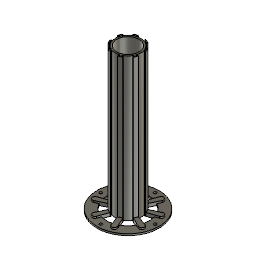
Wifi lamp assembly (Autodesk Fusion 360 archive; units mm, degrees)
design "core lamp comp"
part number: 2026-05-21-12-38-38-254
Autodesk Fusion 360 part; units mm, degrees
sketch "Sketch1" plane through (0, 0, 0) normal (0, 0, 1) x (1, 0, 0)
  circle A0 centre (0, 0) radius 15
  circle A1 centre (0, 0) radius 13
  dimension "d1" = 30
  dimension "d2" = 26
  constraint coincident A0.centre A1.centre
  constraint concentric A0 A1
  measures "d1" diameter of A0
  measures "d2" diameter of A1
extrude "Extrude1" add sketch "Sketch1" along normal blind 168
sketch "Sketch2" plane through (0, 0, 0) normal (0, 0, 1) x (1, 0, 0)
  arc A0 (8.734, 14.7919) -> (4.284, 16.6352) centre (0, 0) ccw
  line L0 (4.284, 16.6352) -> (3.943, 15.6953)
  line L1 (8.734, 14.7919) -> (8.31, 13.8864)
  line L2 (3.943, 15.6953) -> (5.3531, 15.1837)
  line L3 (8.31, 13.8864) -> (6.9516, 14.5226)
  circle A1 centre (0, 0) radius 15
  circle A2 centre (0, 0) radius 13
  circle A3 centre (0, 0) radius 15
  line L4 (5.3531, 15.1837) -> (4.978, 14.1499)
  line L5 (6.9516, 14.5226) -> (6.4848, 13.5258)
  point P0 (4.284, 16.6352)
  point P1 (8.734, 14.7919)
  point P2 (3.943, 15.6953)
  point P3 (8.31, 13.8864)
  dimension "d6" = 4.284
  dimension "d7" = 8.734
  dimension "d8" = 17.178
  dimension "d9" = 17.178
  dimension "d10" = 16.183
  dimension "d11" = 3.943
  dimension "d12" = 16.183
  dimension "d13" = 8.31
  dimension "d14" = 1.5
  dimension "d15" = 1.5
  constraint coincident P1 A0.start
  constraint coincident A0.centre A1.centre
  constraint coincident P0 A0.end
  constraint coincident P2 L0.end
  constraint coincident P3 L1.end
  constraint perpendicular L0 L2
  constraint perpendicular L1 L3
  constraint coincident A1 L4.end
  constraint perpendicular L2 L4
  constraint coincident A1 L5.end
  constraint perpendicular L3 L5
  measures "d6" horizontal distance of A0.centre A0.end
  measures "d7" horizontal distance of A0.centre P1
  measures "d8" distance of A0.centre P1
  measures "d9" distance of A0.centre A0.end
  measures "d10" distance of A0.centre P2
  measures "d11" horizontal distance of A0.centre P2
  measures "d12" distance of A0.centre P3
  measures "d13" horizontal distance of A0.centre P3
  measures "d14" distance of P2 L2.end
  measures "d15" distance of P3 L3.end
extrude "Extrude2" add sketch "Sketch2" along normal blind 168 contours A0 L0 L1 L2 L3 A1 A3 L4 L5
sketch "Sketch3" plane through (0, 0, 0) normal (0, 0, 1) x (1, 0, 0)
  circle A0 centre (11.412, 27.5532) radius 2.99
  circle A1 centre (0, 0) radius 13
  arc A2 (4.978, 14.1499) -> (6.4848, 13.5258) centre (0, 0) ccw
  line L0 (4.978, 14.1499) -> (5.3531, 15.1837)
  line L1 (5.3531, 15.1837) -> (3.943, 15.6953)
  line L2 (3.943, 15.6953) -> (4.284, 16.6352)
  arc A3 (8.734, 14.7919) -> (4.284, 16.6352) centre (0, 0) ccw
  line L3 (8.734, 14.7919) -> (8.31, 13.8864)
  line L4 (8.31, 13.8864) -> (6.9516, 14.5226)
  line L5 (6.9516, 14.5226) -> (6.4848, 13.5258)
  line L6 (8.734, 14.7919) -> (14.1195, 26.2844)
  line L7 (4.284, 16.6352) -> (8.6002, 28.5701)
  dimension "d18" = 5.98
  dimension "d19" = 29.823
  dimension "d20" = 11.412
  constraint coincident A3.start L3.start
  constraint coincident A0 L6.end
  constraint tangent A0 L6
  constraint coincident L2.end A3.end
  constraint coincident A0 L7.end
  constraint tangent A0 L7
  measures "d18" diameter of A0
  measures "d19" distance of A1.centre A0.centre
  measures "d20" horizontal distance of A1.centre A0.centre
extrude "Extrude3" add sketch "Sketch3" along normal blind 4 contours A0 | A0 A3 L6 L7
pattern_circular "C-Pattern1" count 8 over 360 about axis through (0, 0, 1.75) along (0, 0, 1) of "Extrude2", "Extrude3"
sketch "Sketch4" plane through (0, 0, 0) normal (0, 0, 1) x (1, 0, 0)
  circle A0 centre (0, 0) radius 36.6
  circle A1 centre (0, 0) radius 25
  dimension "d25" = 73.2
  dimension "d26" = -11.6
  constraint coincident A0.centre A1.centre
  measures "d25" diameter of A0
extrude "Extrude4" add sketch "Sketch4" along normal blind 2
sketch "Sketch5" plane through (0, 0, 2) normal (0, 0, 1) x (-1, 0, 0)
  circle A0 centre (0, 0) radius 36.6
  line L0 (-21.8965, -12.0642) -> (-26.2834, -14.1208)
  arc A1 (-28.5699, -8.6019) -> (-26.2834, -14.1208) centre (-27.5525, -11.4135) ccw
  line L1 (-28.5699, -8.6019) -> (-24.0136, -6.9533)
  arc A2 (-24.0138, 6.9525) -> (-24.0136, -6.9533) centre (0, 0) ccw
  line L2 (-24.0138, 6.9525) -> (-28.5701, 8.6002)
  arc A3 (-26.2844, 14.1195) -> (-28.5701, 8.6002) centre (-27.5532, 11.412) ccw
  line L3 (-26.2844, 14.1195) -> (-21.8969, 12.0634)
  arc A4 (-12.0642, 21.8965) -> (-21.8969, 12.0634) centre (0, 0) ccw
  line L4 (-12.0642, 21.8965) -> (-14.1208, 26.2834)
  arc A5 (-8.6019, 28.5699) -> (-14.1208, 26.2834) centre (-11.4135, 27.5525) ccw
  line L5 (-8.6019, 28.5699) -> (-6.9533, 24.0136)
  arc A6 (6.9525, 24.0138) -> (-6.9533, 24.0136) centre (0, 0) ccw
  line L6 (6.9525, 24.0138) -> (8.6002, 28.5701)
  arc A7 (14.1195, 26.2844) -> (8.6002, 28.5701) centre (11.412, 27.5532) ccw
  line L7 (14.1195, 26.2844) -> (12.0634, 21.8969)
  arc A8 (21.8965, 12.0642) -> (12.0634, 21.8969) centre (0, 0) ccw
  line L8 (21.8965, 12.0642) -> (26.2834, 14.1208)
  arc A9 (28.5699, 8.6019) -> (26.2834, 14.1208) centre (27.5525, 11.4135) ccw
  line L9 (28.5699, 8.6019) -> (24.0136, 6.9533)
  arc A10 (24.0138, -6.9525) -> (24.0136, 6.9533) centre (0, 0) ccw
  line L10 (24.0138, -6.9525) -> (28.5701, -8.6002)
  arc A11 (26.2844, -14.1195) -> (28.5701, -8.6002) centre (27.5532, -11.412) ccw
  line L11 (26.2844, -14.1195) -> (21.8969, -12.0634)
  arc A12 (12.0642, -21.8965) -> (21.8969, -12.0634) centre (0, 0) ccw
  line L12 (12.0642, -21.8965) -> (14.1208, -26.2834)
  arc A13 (8.6019, -28.5699) -> (14.1208, -26.2834) centre (11.4135, -27.5525) ccw
  line L13 (8.6019, -28.5699) -> (6.9533, -24.0136)
  arc A14 (-6.9525, -24.0138) -> (6.9533, -24.0136) centre (0, 0) ccw
  line L14 (-6.9525, -24.0138) -> (-8.6002, -28.5701)
  arc A15 (-14.1195, -26.2844) -> (-8.6002, -28.5701) centre (-11.412, -27.5532) ccw
  line L15 (-14.1195, -26.2844) -> (-12.0634, -21.8969)
  arc A16 (-21.8965, -12.0642) -> (-12.0634, -21.8969) centre (0, 0) ccw
  circle A17 centre (0, -32) radius 1.6
  dimension "d29" = 3.2
  dimension "d30" = 32
  constraint vertical A0.centre A17.centre
  measures "d29" diameter of A17
  measures "d30" vertical distance of A0.centre A17.centre
extrude "Extrude5" cut sketch "Sketch5" against normal through all contours A17
pattern_circular "C-Pattern2" count 4 over 360 about axis through (0, 0, 1.75) along (0, 0, 1) of "Extrude5"

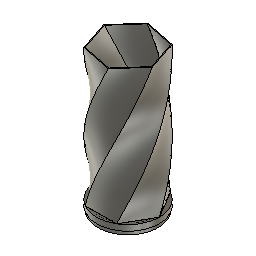
design "LAMP TWISTED HULL"
part number: 2026-05-21-10-49-18-693
Autodesk Fusion 360 part; units mm, degrees
sketch "Sketch1" plane through (0, 0, 0) normal (0, 0, 1) x (1, 0, 0)
  circle A0 centre (0, 0) radius 38.7995
  circle A1 centre (0, 0) radius 36.9995
  dimension "d1" = 77.599
  dimension "d2" = 73.999
  constraint coincident A0.centre A1.centre
  measures "d1" diameter of A0
  measures "d2" diameter of A1
extrude "Extrude1" add sketch "Sketch1" along normal blind 4.8 from surface at 17.9
sketch "Sketch2" plane through (0, 0, 22.7) normal (0, 0, 1) x (-1, 0, 0)
  circle A0 centre (0, 0) radius 36.9995
  circle A1 centre (0, 0) radius 38.7995
  circle A2 centre (0, 0) radius 40
  dimension "d6" = 80
  constraint concentric A0 A2
  measures "d6" diameter of A2
extrude "Extrude2" add sketch "Sketch2" along normal blind 7.3 contours A1 | A2
sketch "Sketch3" plane through (0, 0, 30) normal (0, 0, 1) x (-1, 0, 0)
  circle A0 centre (0, 0) radius 36.9995
  circle A1 centre (0, 0) radius 40
  line L0 (-40, 0) -> (-20, -34.641)
  line L1 (-20, -34.641) -> (20, -34.641)
  line L2 (20, -34.641) -> (40, 0)
  line L3 (40, 0) -> (20, 34.641)
  line L4 (20, 34.641) -> (-20, 34.641)
  line L5 (-20, 34.641) -> (-40, 0)
  line L6 (38.8453, 0) -> (19.4226, 33.641)
  line L7 (19.4226, 33.641) -> (-19.4226, 33.641)
  line L8 (-19.4226, 33.641) -> (-38.8453, 0)
  line L9 (-38.8453, 0) -> (-19.4226, -33.641)
  line L10 (-19.4226, -33.641) -> (19.4226, -33.641)
  line L11 (19.4226, -33.641) -> (38.8453, 0)
  dimension "d9" = 40
  dimension "d10" = 20
  dimension "d11" = -1
  constraint coincident A0.centre A1.centre
  measures "d9" horizontal distance of L3.end L4.end
  measures "d10" horizontal distance of A0.centre L0.end
sketch "Sketch4" plane through (0, 0, 0) normal (0, 1, 0) x (1, 0, 0)
  line L0 (0, -30) -> (0, -200)
  dimension "d12" = 170
  constraint vertical L0
  measures "d12" distance of L0.start L0.end
sweep "Sweep1" add twist angle 108.3 profiles "Sketch3" path "Sketch4" along L0 section 1 contours A0 L3 L6 | A0 L2 L3 L6 L11 | A0 L2 L11 | A0 L3 L4 L6 L7 | A0 L1 L2 L10 L11 | A0 L4 L7 | A0 L1 L10 | A0 L4 L5 L7 L8 | A0 L0 L1 L9 L10 | A0 L5 L8 | A0 L0 L9 | A0 L0 L5 L8 L9
sketch "Sketch5" plane through (0, 0, 30) normal (0, 0, 1) x (-1, 0, 0)
  line L0 (-23.5007, 28.5776) -> (-20, 34.641)
  arc A0 (-20, 34.641) -> (-40, 0) centre (0, 0) ccw
  line L1 (-40, 0) -> (-36.4993, 6.0634)
  arc A1 (-23.5007, 28.5776) -> (-36.4993, 6.0634) centre (0, 0) ccw
  arc A2 (-23.5007, 28.5776) -> (-36.4993, 6.0634) centre (0, 0) ccw
  line L2 (-23.5007, 28.5776) -> (-36.4993, 6.0634)
  point P0 (-36.4993, 6.0634)
  point P1 (-23.5007, 28.5776)
extrude "Extrude3" add sketch "Sketch5" against normal blind 0.8
pattern_circular "C-Pattern1" count 6 over 360 about axis through (0, 0, 1.75) along (0, 0, 1) of "Extrude3"

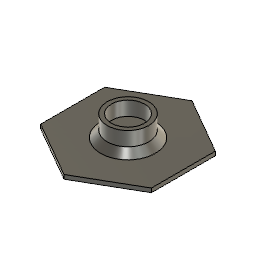
design "WiFi_Controlled_Desk_Lamp_Twisted_Top"
part number: 2026-05-21-09-09-44-045
Autodesk Fusion 360 part; units mm, degrees
sketch "Sketch1" plane through (0, 0, 0) normal (0, 0, 1) x (1, 0, 0)
  line L0 (33.4251, -19.298) -> (33.4251, 19.298)
  line L1 (33.4251, 19.298) -> (0, 38.596)
  line L2 (0, 38.596) -> (-33.4251, 19.298)
  line L3 (-33.4251, 19.298) -> (-33.4251, -19.298)
  line L4 (-33.4251, -19.298) -> (0, -38.596)
  line L5 (0, -38.596) -> (33.4251, -19.298)
  dimension "d1" = 38.596
  constraint vertical origin L1.end
  measures "d1" distance of L1.end origin
extrude "Extrude1" add sketch "Sketch1" along normal blind 2.5
sketch "Sketch2" plane through (0, 0, 2.5) normal (0, 0, 1) x (-1, 0, 0)
  line L0 (0, 38.596) -> (-33.4251, 19.298)
  line L1 (-33.4251, 19.298) -> (-33.4251, -19.298)
  line L2 (-33.4251, -19.298) -> (0, -38.596)
  line L3 (0, -38.596) -> (33.4251, -19.298)
  line L4 (33.4251, -19.298) -> (33.4251, 19.298)
  line L5 (33.4251, 19.298) -> (0, 38.596)
  circle A0 centre (0, 0) radius 16.5
  dimension "d4" = 33
  constraint coincident A0.centre origin
  measures "d4" diameter of A0
extrude "Extrude2" add sketch "Sketch2" along normal blind 4 draft -45 contours A0
sketch "Sketch3" plane through (0, 0, 6.5) normal (0, 0, 1) x (-1, 0, 0)
  circle A0 centre (0, 0) radius 12.5
  circle A1 centre (0, 0) radius 10
  dimension "d7" = 20
  constraint coincident A0.centre A1.centre
  measures "d7" diameter of A1
extrude "Extrude3" add sketch "Sketch3" along normal blind 8.5

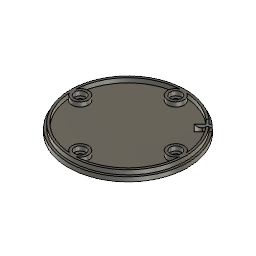
design "Wifi_top_cover"
part number: 2026-05-21-09-43-14-642
Autodesk Fusion 360 part; units mm, degrees
sketch "Sketch1" plane through (0, 0, 0) normal (0, 0, 1) x (1, 0, 0)
  circle A0 centre (0, 0) radius 40
  dimension "d1" = 80
  constraint coincident A0.centre origin
  measures "d1" diameter of A0
extrude "Extrude1" add sketch "Sketch1" along normal blind 3
sketch "Sketch2" plane through (0, 0, 3) normal (0, 0, 1) x (-1, 0, 0)
  circle A0 centre (0, 0) radius 40
  circle A1 centre (0, 0) radius 38.5
  circle A2 centre (0, 32) radius 3.75
  circle A3 centre (0, 32) radius 5.5
  circle A4 centre (0, 0) radius 37
  dimension "d4" = 77
  dimension "d5" = 7.5
  dimension "d6" = 11
  dimension "d7" = 32
  dimension "d8" = 74
  constraint coincident A0.centre A1.centre
  constraint concentric A2 A3
  measures "d4" diameter of A1
  measures "d5" diameter of A2
  measures "d6" diameter of A3
  measures "d7" distance of A0.centre A2.centre
  measures "d8" diameter of A4
extrude "Extrude2" add sketch "Sketch2" along normal blind 3 contours A1 | A3 A4 | A3 A4 picked at (-1.5513, 36.4665) picked at (0.1215, 37.1566)
pattern_circular "C-Pattern1" count 4 over 360 about axis through (0, 0, 1.75) along (0, 0, 1) of "Extrude2"
sketch "Sketch3" plane through (0, 0, 0) normal (0, 0, -1) x (1, 0, 0)
  circle A0 centre (0, 0) radius 40
  circle A1 centre (0, -32) radius 3
  dimension "d13" = 6
  dimension "d14" = 32
  measures "d13" diameter of A1
  measures "d14" distance of A0.centre A1.centre
extrude "Extrude3" cut sketch "Sketch3" against normal through all draft -25 contours A1
pattern_circular "C-Pattern2" count 4 over 360 about axis through (0, 0, 0) along (0, 0, 1) of "Extrude3"
ref_plane "WorkPlane1" through (0, 0, 0) normal (-0.707107, 0.707107, 0) x (0, 0, 1)
sketch "Sketch4" plane through (0, 0, 0) normal (-0.707107, 0.707107, 0) x (0, 0, 1)
  line L0 (6, -27.2236) -> (6, 38.5)
  line L1 (6, -38.5) -> (6, -27.2236)
  line L2 (3, -40) -> (3, -38.5)
  line L3 (3, 38.5) -> (3, 40)
  line L4 (0, -40) -> (0, 40)
  line L5 (3, -38.5) -> (6, -38.5)
  line L6 (3, 38.5) -> (6, 38.5)
  line L7 (0, -40) -> (3, -40)
  line L8 (0, 40) -> (3, 40)
  line L9 (3, 40) -> (6, 40)
  line L10 (6, 40) -> (6, 30.653)
  line L11 (3, 40) -> (1, 40)
  line L12 (1, 40) -> (1, 35.115)
  arc A0 (1, 35.115) -> (6, 30.653) centre (5.4909, 35.115) ccw
  dimension "d18" = 3
  dimension "d19" = 9.347
  dimension "d20" = 2
  dimension "d21" = 4.885
  constraint coincident L3.end L8.end
  constraint perpendicular L3 L9
  constraint perpendicular L9 L10
  constraint perpendicular L3 L11
  constraint perpendicular L11 L12
  constraint tangent L12 A0
  measures "d18" distance of L3.end L9.end
  measures "d19" distance of L9.end L10.end
  measures "d20" distance of L3.end L11.end
  measures "d21" distance of L11.end L12.end
extrude "Extrude4" cut sketch "Sketch4" along normal mid plane 6 contours L0 L3 L6 L8 L10 L11 L12 A0 | L3 L6 L9 L10

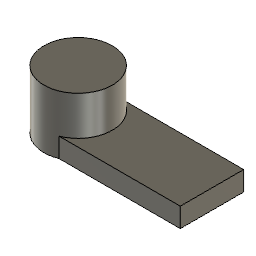
design "WiFi_Controlled_Desk_Lamp_Button"
part number: 2026-05-21-09-30-18-419
Autodesk Fusion 360 part; units mm, degrees
sketch "Sketch1" plane through (0, 0, 0) normal (0, 0, 1) x (1, 0, 0)
  circle A0 centre (0, 0) radius 3.5
  dimension "d1" = 7
  constraint coincident A0.centre origin
  measures "d1" diameter of A0
extrude "Extrude1" add sketch "Sketch1" along normal blind 6
sketch "Sketch2" plane through (0, 0, 0) normal (0, 0, 1) x (1, 0, 0)
  line L0 (0, 3.25) -> (13.701, 3.25)
  line L1 (13.701, 3.25) -> (13.701, -3.25)
  line L2 (13.701, -3.25) -> (0, -3.25)
  line L3 (0, -3.25) -> (0, 3.25)
  dimension "d4" = 6.5
  dimension "d5" = 13.701
  constraint horizontal L0
  constraint vertical L1
  constraint horizontal L2
  constraint vertical L3
  constraint midpoint origin L3
  measures "d4" distance of L0.start L2.end
  measures "d5" distance of L1.end L2.end
extrude "Extrude2" add sketch "Sketch2" along normal blind 2
